Autodesk Fusion 360 part; units mm, degrees
(part 3 of 3)
sketch "Sketch6" plane through (0, 0, 4.8) normal (0, 0, 1) x (-1, 0, 0)
  circle A0 centre (64.2941, -62.4) radius 1.5
  circle A1 centre (64.2941, 62.4) radius 1.5
  circle A2 centre (97.2941, -62.4) radius 1.5
  circle A3 centre (97.2941, 62.4) radius 1.5
  circle A4 centre (1.7941, -104.2) radius 6.1
  line L0 (15.4941, 111.4) -> (41.8941, 111.4)
  arc A5 (45.5941, 107.7) -> (41.8941, 111.4) centre (41.8941, 107.7) ccw
  line L1 (45.5941, 107.7) -> (45.5941, 100.7)
  arc A6 (41.8941, 97) -> (45.5941, 100.7) centre (41.8941, 100.7) ccw
  line L2 (41.8941, 97) -> (15.4941, 97)
  arc A7 (11.7941, 100.7) -> (15.4941, 97) centre (15.4941, 100.7) ccw
  line L3 (11.7941, 100.7) -> (11.7941, 107.7)
  arc A8 (15.4941, 111.4) -> (11.7941, 107.7) centre (15.4941, 107.7) ccw
  line L4 (15.4941, -97) -> (41.8941, -97)
  arc A9 (45.5941, -100.7) -> (41.8941, -97) centre (41.8941, -100.7) ccw
  line L5 (45.5941, -100.7) -> (45.5941, -107.7)
  arc A10 (41.8941, -111.4) -> (45.5941, -107.7) centre (41.8941, -107.7) ccw
  line L6 (41.8941, -111.4) -> (15.4941, -111.4)
  arc A11 (11.7941, -107.7) -> (15.4941, -111.4) centre (15.4941, -107.7) ccw
  line L7 (11.7941, -107.7) -> (11.7941, -100.7)
  arc A12 (15.4941, -97) -> (11.7941, -100.7) centre (15.4941, -100.7) ccw
  circle A13 centre (45.4941, 42.5) radius 1.5
  line L8 (48.7941, 89.8787) -> (48.7941, 87.5)
  arc A14 (48.7941, 87.5) -> (50.2941, 86) centre (50.2941, 87.5) ccw
  line L9 (50.2941, 86) -> (55.6728, 86)
  arc A15 (57.7941, 83.8787) -> (55.6728, 86) centre (56.7335, 84.9393) ccw
  line L10 (57.7941, 83.8787) -> (57.7941, 58.1213)
  arc A16 (55.6728, 56) -> (57.7941, 58.1213) centre (56.7335, 57.0607) ccw
  line L11 (55.6728, 56) -> (13.9155, 56)
  arc A17 (11.7941, 58.1213) -> (13.9155, 56) centre (12.8548, 57.0607) ccw
  line L12 (11.7941, 58.1213) -> (11.7941, 89.8787)
  arc A18 (13.9155, 92) -> (11.7941, 89.8787) centre (12.8548, 90.9393) ccw
  line L13 (13.9155, 92) -> (46.6728, 92)
  arc A19 (48.7941, 89.8787) -> (46.6728, 92) centre (47.7335, 90.9393) ccw
  arc A20 (94.6728, -10) -> (96.7941, -7.8787) centre (95.7335, -8.9393) ccw
  line L14 (94.6728, -10) -> (94.1155, -10)
  arc A21 (91.9941, -7.8787) -> (94.1155, -10) centre (93.0548, -8.9393) ccw
  line L15 (91.9941, -7.8787) -> (91.9941, 7.8787)
  arc A22 (94.1155, 10) -> (91.9941, 7.8787) centre (93.0548, 8.9393) ccw
  line L16 (94.1155, 10) -> (94.6728, 10)
  arc A23 (96.7941, 7.8787) -> (94.6728, 10) centre (95.7335, 8.9393) ccw
  line L17 (96.7941, 7.8787) -> (96.7941, -7.8787)
  arc A24 (39.8728, -10) -> (41.9941, -7.8787) centre (40.9335, -8.9393) ccw
  line L18 (39.8728, -10) -> (39.3155, -10)
  arc A25 (37.1941, -7.8787) -> (39.3155, -10) centre (38.2548, -8.9393) ccw
  line L19 (37.1941, -7.8787) -> (37.1941, 7.8787)
  arc A26 (39.3155, 10) -> (37.1941, 7.8787) centre (38.2548, 8.9393) ccw
  line L20 (39.3155, 10) -> (39.8728, 10)
  arc A27 (41.9941, 7.8787) -> (39.8728, 10) centre (40.9335, 8.9393) ccw
  line L21 (41.9941, 7.8787) -> (41.9941, -7.8787)
  circle A28 centre (-123.5112, 37.2289) radius 1.5
  circle A29 centre (64.5, 111.7173) radius 1.5
  arc A30 (-55.2202, 79.8868) -> (-55.9967, 76.9891) centre (-55.6084, 78.438) ccw
  line L22 (-55.2202, 79.8868) -> (-41.5739, 87.7655)
  arc A31 (-38.6762, 86.9891) -> (-41.5739, 87.7655) centre (-40.125, 87.3773) ccw
  line L23 (-38.6762, 86.9891) -> (-38.3975, 86.5064)
  arc A32 (-39.1739, 83.6086) -> (-38.3975, 86.5064) centre (-38.7857, 85.0575) ccw
  line L24 (-39.1739, 83.6086) -> (-52.8202, 75.7299)
  arc A33 (-55.718, 76.5064) -> (-52.8202, 75.7299) centre (-54.2691, 76.1181) ccw
  line L25 (-55.718, 76.5064) -> (-55.9967, 76.9891)
  circle A34 centre (-123.5112, -37.2289) radius 1.5
  circle A35 centre (64.5, -111.7173) radius 1.5
  arc A36 (-11.2762, 39.5309) -> (-14.1739, 40.3073) centre (-12.725, 39.9191) ccw
  line L26 (-11.2762, 39.5309) -> (-10.9975, 39.0482)
  arc A37 (-11.7739, 36.1504) -> (-10.9975, 39.0482) centre (-11.3857, 37.5993) ccw
  line L27 (-11.7739, 36.1504) -> (-25.4202, 28.2717)
  arc A38 (-28.318, 29.0482) -> (-25.4202, 28.2717) centre (-26.8691, 28.66) ccw
  line L28 (-28.318, 29.0482) -> (-28.5967, 29.5309)
  arc A39 (-27.8202, 32.4286) -> (-28.5967, 29.5309) centre (-28.2084, 30.9798) ccw
  line L29 (-27.8202, 32.4286) -> (-14.1739, 40.3073)
  arc A40 (-10.9975, -39.0482) -> (-11.7739, -36.1504) centre (-11.3857, -37.5993) ccw
  line L30 (-10.9975, -39.0482) -> (-11.2762, -39.5309)
  arc A41 (-14.1739, -40.3073) -> (-11.2762, -39.5309) centre (-12.725, -39.9191) ccw
  line L31 (-14.1739, -40.3073) -> (-27.8202, -32.4286)
  arc A42 (-28.5967, -29.5309) -> (-27.8202, -32.4286) centre (-28.2084, -30.9798) ccw
  line L32 (-28.5967, -29.5309) -> (-28.318, -29.0482)
  arc A43 (-25.4202, -28.2717) -> (-28.318, -29.0482) centre (-26.8691, -28.66) ccw
  line L33 (-25.4202, -28.2717) -> (-11.7739, -36.1504)
  line L34 (55.6728, -86) -> (50.2941, -86)
  arc A44 (50.2941, -86) -> (48.7941, -87.5) centre (50.2941, -87.5) ccw
  line L35 (48.7941, -87.5) -> (48.7941, -89.8787)
  arc A45 (46.6728, -92) -> (48.7941, -89.8787) centre (47.7335, -90.9393) ccw
  line L36 (46.6728, -92) -> (13.9155, -92)
  arc A46 (11.7941, -89.8787) -> (13.9155, -92) centre (12.8548, -90.9393) ccw
  line L37 (11.7941, -89.8787) -> (11.7941, -58.1213)
  arc A47 (13.9155, -56) -> (11.7941, -58.1213) centre (12.8548, -57.0607) ccw
  line L38 (13.9155, -56) -> (55.6728, -56)
  arc A48 (57.7941, -58.1213) -> (55.6728, -56) centre (56.7335, -57.0607) ccw
  line L39 (57.7941, -58.1213) -> (57.7941, -83.8787)
  arc A49 (55.6728, -86) -> (57.7941, -83.8787) centre (56.7335, -84.9393) ccw
  arc A50 (-52.8202, -75.7299) -> (-55.718, -76.5064) centre (-54.2691, -76.1181) ccw
  line L40 (-52.8202, -75.7299) -> (-39.1739, -83.6086)
  arc A51 (-38.3975, -86.5064) -> (-39.1739, -83.6086) centre (-38.7857, -85.0575) ccw
  line L41 (-38.3975, -86.5064) -> (-38.6762, -86.9891)
  arc A52 (-41.5739, -87.7655) -> (-38.6762, -86.9891) centre (-40.125, -87.3773) ccw
  line L42 (-41.5739, -87.7655) -> (-55.2202, -79.8868)
  arc A53 (-55.9967, -76.9891) -> (-55.2202, -79.8868) centre (-55.6084, -78.438) ccw
  line L43 (-55.9967, -76.9891) -> (-55.718, -76.5064)
  circle A54 centre (45.4941, -42.5) radius 1.5
  line L44 (-42.1213, -25.5) -> (-109.5263, -25.5)
  arc A55 (-109.5263, -25.5) -> (-110.7763, -25.8349) centre (-109.5263, -28) ccw
  line L45 (-110.7763, -25.8349) -> (-125.9451, -34.5927)
  arc A56 (-125.9451, -34.5927) -> (-127.0931, -37.4646) centre (-124.6951, -36.7577) ccw
  arc A57 (-127.0931, -37.4646) -> (-89.0244, -98.1371) centre (0, 0) ccw
  arc A58 (-89.0244, -98.1371) -> (-85.1797, -97.5355) centre (-87.3447, -96.2855) ccw
  line L46 (-85.1797, -97.5355) -> (-74.6084, -79.2255)
  arc A59 (-71.7106, -78.449) -> (-74.6084, -79.2255) centre (-73.1595, -78.8372) ccw
  line L47 (-71.7106, -78.449) -> (-32.0836, -101.3277)
  arc A60 (-31.3071, -104.2255) -> (-32.0836, -101.3277) centre (-31.6953, -102.7766) ccw
  line L48 (-31.3071, -104.2255) -> (-41.8784, -122.5355)
  arc A61 (-41.8784, -122.5355) -> (-40.477, -126.166) centre (-39.7133, -123.7855) ccw
  arc A62 (-40.477, -126.166) -> (129.5015, -28.0288) centre (0, 0) ccw
  arc A63 (129.5015, -28.0288) -> (127.0581, -25) centre (127.0581, -27.5) ccw
  line L49 (127.0581, -25) -> (105.9155, -25)
  arc A64 (103.7941, -22.8787) -> (105.9155, -25) centre (104.8548, -23.9393) ccw
  line L50 (103.7941, -22.8787) -> (103.7941, 22.8787)
  arc A65 (105.9155, 25) -> (103.7941, 22.8787) centre (104.8548, 23.9393) ccw
  line L51 (105.9155, 25) -> (127.0581, 25)
  arc A66 (127.0581, 25) -> (129.5015, 28.0288) centre (127.0581, 27.5) ccw
  arc A67 (129.5015, 28.0288) -> (-40.477, 126.166) centre (0, 0) ccw
  arc A68 (-40.477, 126.166) -> (-41.8784, 122.5355) centre (-39.7133, 123.7855) ccw
  line L52 (-41.8784, 122.5355) -> (-31.3071, 104.2255)
  arc A69 (-32.0836, 101.3277) -> (-31.3071, 104.2255) centre (-31.6953, 102.7766) ccw
  line L53 (-32.0836, 101.3277) -> (-71.7106, 78.449)
  arc A70 (-74.6084, 79.2255) -> (-71.7106, 78.449) centre (-73.1595, 78.8372) ccw
  line L54 (-74.6084, 79.2255) -> (-85.1797, 97.5355)
  arc A71 (-85.1797, 97.5355) -> (-89.0244, 98.1371) centre (-87.3447, 96.2855) ccw
  arc A72 (-89.0244, 98.1371) -> (-127.0931, 37.4646) centre (0, 0) ccw
  arc A73 (-127.0931, 37.4646) -> (-125.9451, 34.5927) centre (-124.6951, 36.7577) ccw
  line L55 (-125.9451, 34.5927) -> (-110.7763, 25.8349)
  arc A74 (-110.7763, 25.8349) -> (-109.5263, 25.5) centre (-109.5263, 28) ccw
  line L56 (-109.5263, 25.5) -> (-42.1213, 25.5)
  arc A75 (-40, 23.3787) -> (-42.1213, 25.5) centre (-41.0607, 24.4393) ccw
  line L57 (-40, 23.3787) -> (-40, 20.8)
  arc A76 (-40, 20.8) -> (-37.5, 18.3) centre (-37.5, 20.8) ccw
  line L58 (-37.5, 18.3) -> (-34.1213, 18.3)
  arc A77 (-32, 16.1787) -> (-34.1213, 18.3) centre (-33.0607, 17.2393) ccw
  line L59 (-32, 16.1787) -> (-32, -16.1787)
  arc A78 (-34.1213, -18.3) -> (-32, -16.1787) centre (-33.0607, -17.2393) ccw
  line L60 (-34.1213, -18.3) -> (-37.5, -18.3)
  arc A79 (-37.5, -18.3) -> (-40, -20.8) centre (-37.5, -20.8) ccw
  line L61 (-40, -20.8) -> (-40, -23.3787)
  arc A80 (-42.1213, -25.5) -> (-40, -23.3787) centre (-41.0607, -24.4393) ccw
  arc A81 (-40.477, -126.166) -> (129.5015, -28.0288) centre (0, 0) ccw
  line L62 (57.7941, -64.8) -> (103.7941, -64.8)
  line L63 (57.7941, -58.1213) -> (57.7941, -83.8787)
  arc A82 (129.5015, 28.0288) -> (-40.477, 126.166) centre (0, 0) ccw
  line L64 (57.7941, 64.8) -> (103.7941, 64.8)
  line L65 (57.7941, 58.1213) -> (57.7941, 83.8787)
  line L66 (95.1844, -72.8) -> (67.2941, -72.8)
  line L67 (65.7941, -74.3) -> (65.7941, -100.26)
  arc A83 (68.1301, -101.5054) -> (96.3668, -75.223) centre (0, 0) ccw
  arc A84 (67.2941, -72.8) -> (65.7941, -74.3) centre (67.2941, -74.3) ccw
  arc A85 (65.7941, -100.26) -> (68.1301, -101.5054) centre (67.2941, -100.26) ccw
  arc A86 (96.3668, -75.223) -> (95.1844, -72.8) centre (95.1844, -74.3) ccw
  line L68 (95.1844, 72.8) -> (67.2941, 72.8)
  line L69 (65.7941, 74.3) -> (65.7941, 100.26)
  arc A87 (96.3668, 75.223) -> (68.1301, 101.5054) centre (0, 0) ccw
  arc A88 (65.7941, 74.3) -> (67.2941, 72.8) centre (67.2941, 74.3) ccw
  arc A89 (95.1844, 72.8) -> (96.3668, 75.223) centre (95.1844, 74.3) ccw
  arc A90 (68.1301, 101.5054) -> (65.7941, 100.26) centre (67.2941, 100.26) ccw
  dimension "d304" = 8
  dimension "d305" = 8
  dimension "d306" = 122.25
  dimension "d307" = 1.5
  dimension "d308" = 1.5
  dimension "d309" = 1.5
  dimension "d310" = 8
  dimension "d311" = 8
  dimension "d312" = 122.25
  dimension "d313" = 1.5
  dimension "d314" = 1.5
  dimension "d315" = 1.5
  constraint perpendicular L63 L66
  constraint perpendicular L66 L67
  constraint coincident A57.centre A62.centre
  constraint tangent L66 A84
  constraint tangent L67 A84
  constraint tangent A83 A85
  constraint tangent L67 A85
  constraint tangent A83 A86
  constraint tangent L66 A86
  constraint perpendicular L65 L68
  constraint perpendicular L68 L69
  constraint tangent L68 A88
  constraint tangent L69 A88
  constraint tangent A87 A89
  constraint tangent L68 A89
  constraint tangent A87 A90
  constraint tangent L69 A90
  measures "d304" distance of L62 L66
  measures "d305" distance of L63 L67
  measures "d306" radius of A83
  measures "d307" radius of A84
  measures "d308" radius of A85
  measures "d309" radius of A86
  measures "d310" distance of L64 L68
  measures "d311" distance of L65 L69
  measures "d312" radius of A87
  measures "d313" radius of A88
  measures "d314" radius of A89
  measures "d315" radius of A90
extrude "Extrude9" cut sketch "Sketch6" against normal through all contours L66 L67 A83 A84 A85 A86 | L68 L69 A87 A88 A89 A90
